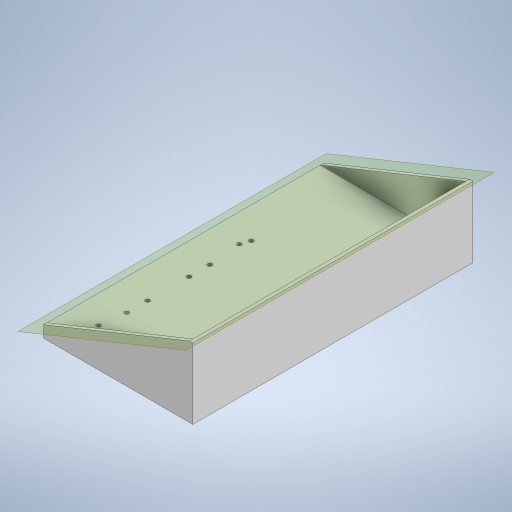
# Autodesk Inventor part: Soporte
Saved by Autodesk Inventor 2023 (Build 270158000, 158)
## iProperties
Created: 2024-01-17
Part Number: Soporte
Material: Generic
Document SubType Name: Modeling
Designer: juanp
Density: 1 g/cm^3
Appearance: Default
Author: juanp
Autodesk Inventor part; units mm, degrees
ref_plane "YZ Plane" through (0, 0, 0) normal (1, 0, 0) x (0, 1, 0)
ref_plane "XZ Plane" through (0, 0, 0) normal (0, 1, 0) x (-1, 0, 0)
ref_plane "XY Plane" through (0, 0, 0) normal (0, 0, 1) x (1, 0, 0)
sketch "Sketch1" plane through (0, 0, 0) normal (0, 1, 0) x (-1, 0, 0)
  line L0 (60.5, -116.25) -> (-60.5, -116.25)
  line L1 (-60.5, -116.25) -> (-60.5, 116.25)
  line L2 (-60.5, 116.25) -> (60.5, 116.25)
  line L3 (60.5, 116.25) -> (60.5, -116.25)
  line L4 (60.5, -116.25) -> (-60.5, 116.25) construction
  line L5 (-60.5, -116.25) -> (60.5, 116.25) construction
  line L6 (-40, 10.25) -> (-40, 60.25)
  line L7 (40, 10.25) -> (-40, 10.25)
  line L8 (40, 60.25) -> (40, 10.25)
  line L9 (-40, 60.25) -> (40, 60.25)
  circle A0 centre (37, 22) radius 1.75
  circle A1 centre (-37, 13.25) radius 1.75
  circle A2 centre (37, 57.25) radius 1.75
  circle A3 centre (-37, 57.25) radius 1.75
  circle A4 centre (37, -31) radius 1.75
  line L10 (40, -42.75) -> (-40, -42.75)
  circle A5 centre (-37, -39.75) radius 1.75
  circle A6 centre (37, 4.25) radius 1.75
  line L11 (40, 7.25) -> (40, -42.75)
  line L12 (-40, 7.25) -> (40, 7.25)
  circle A7 centre (-37, 4.25) radius 1.75
  line L13 (-40, -42.75) -> (-40, 7.25)
  circle A8 centre (37, 75) radius 1.75
  line L14 (40, 63.25) -> (-40, 63.25)
  circle A9 centre (-37, 66.25) radius 1.75
  circle A10 centre (37, 110.25) radius 1.75
  line L15 (40, 113.25) -> (40, 63.25)
  line L16 (-40, 113.25) -> (40, 113.25)
  circle A11 centre (-37, 110.25) radius 1.75
  line L17 (-40, 63.25) -> (-40, 113.25)
  line L18 (57.5, -45.75) -> (-57.5, -45.75)
  line L19 (-57.5, -45.75) -> (-57.5, -113.25)
  line L20 (-57.5, -113.25) -> (57.5, -113.25)
  line L21 (57.5, -113.25) -> (57.5, -45.75)
  line L22 (57.5, -45.75) -> (-57.5, -113.25) construction
  line L23 (-57.5, -45.75) -> (57.5, -113.25) construction
  line L24 (0, 113.25) -> (0, 113.2503) construction
  line L25 (63.5, 119.25) -> (-63.5, 119.25)
  line L26 (-63.5, 119.25) -> (-63.5, -119.25)
  line L27 (-63.5, -119.25) -> (63.5, -119.25)
  line L28 (63.5, -119.25) -> (63.5, 119.25)
  point P0 (0, 0)
  point P1 (0, -79.5)
  point P2 (0, -42.75)
  dimension "d6" = 3
  dimension "d7" = 3
  dimension "d8" = 3
  dimension "d9" = 3
  dimension "d10" = 3
  dimension "d11" = 11.75
  dimension "d12" = 3
  dimension "d13" = 3
  dimension "d14" = 50
  dimension "d15" = 80
  dimension "d16" = 3
  dimension "d17" = 3
  dimension "d18" = 3
  dimension "d19" = 3
  dimension "d20" = 3
  dimension "d21" = 11.75
  dimension "d22" = 3
  dimension "d23" = 3
  dimension "d24" = 50
  dimension "d25" = 80
  dimension "d26" = 3
  dimension "d27" = 3
  dimension "d28" = 3
  dimension "d29" = 3
  dimension "d30" = 3
  dimension "d31" = 11.75
  dimension "d32" = 3
  dimension "d33" = 3
  dimension "d34" = 50
  dimension "d35" = 80
  dimension "d36" = 3
  dimension "d37" = 3
  dimension "d38" = 67.5
  dimension "d39" = 115
  dimension "d43" = 3
  dimension "d44" = 3
  dimension "d46" = 3.5
  dimension "d47" = 3
  dimension "d48" = 3
  dimension "d49" = 3
  dimension "d50" = 3
  constraints: 58 end point, 12 centre point, 12 perpendicular, 11 equal radius, 6 midpoint, 6 parallel, 5 horizontal, 2 collinear, 1 point on line, 1 vertical, 3 other
  measures "d6" distance from line of L6 A1.centre
  measures "d7" distance from line of L6 A3.centre
  measures "d8" distance from line of L8 A0.centre
  measures "d9" distance from line of A2.centre L8
  measures "d10" distance from line of L9 A2.centre
  measures "d11" distance from line of L7 A0.centre
  measures "d12" distance from line of L9 A3.centre
  measures "d13" distance from line of L7 A1.centre
  measures "d14" distance of L7.end L9.start
  measures "d15" distance of L9.start L8.start
  measures "d16" distance from line of L13 A5.centre
  measures "d17" distance from line of L13 A7.centre
  measures "d18" distance from line of L11 A4.centre
  measures "d19" distance from line of A6.centre L11
  measures "d20" distance from line of L12 A6.centre
  measures "d21" distance from line of L10 A4.centre
  measures "d22" distance from line of L12 A7.centre
  measures "d23" distance from line of L10 A5.centre
  measures "d24" distance of L13.start L13.end
  measures "d25" distance of L13.end L11.start
  measures "d26" distance from line of L17 A9.centre
  measures "d27" distance from line of L17 A11.centre
  measures "d28" distance from line of L15 A8.centre
  measures "d29" distance from line of A10.centre L15
  measures "d30" distance from line of L16 A10.centre
  measures "d31" distance from line of L14 A8.centre
  measures "d32" distance from line of L16 A11.centre
  measures "d33" distance from line of L14 A9.centre
  measures "d34" distance of L17.start L17.end
  measures "d35" distance of L17.end L15.start
  measures "d36" distance between parallel lines of L9 L14
  measures "d37" distance between parallel lines of L12 L7
  measures "d38" distance of L19.end L18.end
  measures "d39" distance between parallel lines of L19 L21
  measures "d43" distance between parallel lines of L3 L21
  measures "d44" distance between parallel lines of L19 L1
  measures "d46" diameter of A10
  measures "d47" distance between parallel lines of L2 L16
  measures "d48" distance between parallel lines of L0 L20
  measures "d49" distance between parallel lines of L10 L18
  measures "d50" distance between parallel lines of L27 L0
extrude "Extrusion1" add sketch "Sketch1" along normal blind 5 contours L0 L1 L2 L3 | L6 L9 L8 L7 | L10 L13 L12 L11 | L14 L17 L16 L15 | L21 L20 L19 L18 | L28 L27 L26 L25
extrude "Extrusion2" add sketch "Sketch1" against normal blind 5 contours L28 L27 L26 L25
sketch "Sketch2" plane through (0, 0, 0) normal (0, -1, 0) x (1, 0, 0)
  line L0 (-39.6, -23.468) -> (40.4, -23.468) construction
  line L1 (40.4, -23.468) -> (40.4, 96.532) construction
  line L2 (40.4, 96.532) -> (-39.6, 96.532) construction
  line L3 (-39.6, 96.532) -> (-39.6, -23.468) construction
  line L4 (-39.6, -23.468) -> (40.4, 96.532) construction
  line L5 (40.4, -23.468) -> (-39.6, 96.532) construction
  line L6 (-48.6, -83.468) -> (48.6, -83.468) construction
  line L7 (48.6, -83.468) -> (48.6, 115.032) construction
  line L8 (48.6, 115.032) -> (-48.6, 115.032) construction
  line L9 (-48.6, 115.032) -> (-48.6, -83.468) construction
  line L10 (-48.6, -83.468) -> (48.6, 115.032) construction
  line L11 (48.6, -83.468) -> (-48.6, 115.032) construction
  circle A0 centre (-39.6, 96.532) radius 1.65
  circle A1 centre (40.4, 96.532) radius 1.65
  circle A2 centre (40.4, -23.468) radius 1.65
  circle A3 centre (-39.6, -23.468) radius 1.65
  line L12 (60.5, -116.25) -> (-60.5, -116.25) projected
  line L13 (0, -116.25) -> (0, 15.782)
  point P0 (0.4, 36.532)
  point P1 (-39.6, 36.532)
  dimension "d61" = 80
  dimension "d62" = 120
  dimension "d63" = 97.2
  dimension "d64" = 198.5
  dimension "d65" = 9
  dimension "d66" = 60
  dimension "d67" = 3.3
  dimension "d70" = 132.032
  constraints: 26 end point, 6 midpoint, 4 centre point, 4 coincident, 4 parallel, 3 equal radius, 3 perpendicular, 1 horizontal
  measures "d61" distance of L3.start L2.start
  measures "d62" distance of L2.start L0.end
  measures "d63" distance of L9.start L7.end
  measures "d64" distance of L7.end L6.end
  measures "d65" distance from line of L9 point (-39.6, 36.532)
  measures "d66" distance between parallel lines of L6 L0
  measures "d67" diameter of A0
  measures "d70" distance of L13.start L13.end
extrude "Extrusion3" cut sketch "Sketch2" against normal blind 5
sketch "Sketch3" plane through (0, 5, 0) normal (0, 1, 0) x (1, 0, 0)
  line L0 (-63.5, -119.25) -> (63.5, -119.25) projected
  line L1 (63.5, 119.25) -> (-63.5, 119.25) projected
  line L2 (63.5, -119.25) -> (60.5, -119.25)
  line L3 (60.5, -119.25) -> (60.5, 119.25)
  line L4 (60.5, 119.25) -> (63.5, 119.25)
  line L5 (63.5, 119.25) -> (63.5, -119.25)
  point P0 (0, 0)
  dimension "d73" = 3
  constraints: 8 end point, 2 parallel, 1 horizontal, 1 perpendicular, 1 point on line
  measures "d73" distance between parallel lines of L5 L3
extrude "Extrusion4" add sketch "Sketch3" along normal blind 50
ref_plane "Work Plane1" through (60.5, 55, -119.25) normal (0.3739683, -0.9274415, 0) x (0, 0, 1)
sketch "Sketch4" plane through (60.5, 55, -119.25) normal (0.3739683, -0.9274415, 0) x (0, 0, 1)
  line L0 (0, 0) -> (238.5, 0) projected
  line L1 (0, 133.7012) -> (238.5, 133.7012) projected
  line L2 (238.5, 0) -> (235.5, 0)
  line L3 (235.5, 0) -> (235.5, 133.7012)
  line L4 (235.5, 133.7012) -> (238.5, 133.7012)
  line L5 (238.5, 133.7012) -> (238.5, 0)
  line L6 (0, -2.7823) -> (0, 0) projected
  line L7 (0, 0) -> (3, 0)
  line L8 (3, 0) -> (3, 133.7012)
  line L9 (3, 133.7012) -> (0, 133.7012)
  line L10 (0, 133.7012) -> (0, 0)
  point P0 (119.25, 76.6785)
  point P1 (0, 133.7012)
  point P2 (238.5, 133.7012)
  point P3 (235.5, 0)
  dimension "d76" = 3
  dimension "d77" = 3
  constraints: 16 end point, 4 parallel, 2 horizontal, 2 perpendicular, 2 point on line
  measures "d76" distance between parallel lines of L5 L3
  measures "d77" distance between parallel lines of L8 L10
extrude "Extrusion5" add sketch "Sketch4" along normal up to next contours L10 L1 L8 L0 | L3 L1 L5 L0
body "Solid1"
